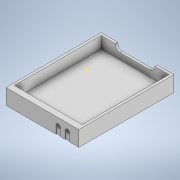
# Autodesk Inventor part: battery-holder-v2
Saved by Autodesk Inventor 2021.2 (Build 252289000, 289)
## iProperties
Created: 2021-03-31
Part Number: battery-holder-v2
Material: Generic
Document SubType Name: Modeling
Designer: ruby
Density: 1 g/cm^3
Appearance: Default
Author: ruby
Autodesk Inventor part; units mm, degrees
ref_plane "YZ Plane" through (0, 0, 0) normal (1, 0, 0) x (0, 1, 0)
ref_plane "XZ Plane" through (0, 0, 0) normal (0, 1, 0) x (-1, 0, 0)
ref_plane "XY Plane" through (0, 0, 0) normal (0, 0, 1) x (1, 0, 0)
sketch "Sketch2" plane through (0, 0, 0) normal (0, 1, 0) x (-1, 0, 0)
  line L0 (11.092548, -17.745585) -> (-22.307452, -17.745585)
  line L1 (-22.307452, -17.745585) -> (-22.307452, 24.254415)
  line L2 (-22.307452, 24.254415) -> (11.092548, 24.254415)
  line L3 (11.092548, 24.254415) -> (11.092548, -17.745585)
  point P0 (0, 0)
  dimension "d2" = 42
  dimension "d3" = 33.4
  constraints: 8 end point, 2 parallel, 1 horizontal, 1 perpendicular
  measures "d2" distance of L2.end L0.start
  measures "d3" distance of L0.start L0.end
sketch "Sketch2 outline for Extrusion1" plane through (0, 0, 0) normal (0, 1, 0) x (-1, 0, 0)
  line L0 (11.092548, -17.745585) -> (11.092548, 24.254415)
  line L1 (-22.307452, -17.745585) -> (11.092548, -17.745585)
  line L2 (-22.307452, 24.254415) -> (-22.307452, -17.745585)
  line L3 (11.092548, 24.254415) -> (-22.307452, 24.254415)
extrude "Extrusion1" add sketch "Sketch2 outline for Extrusion1" along normal blind 6
sketch "Sketch3" plane through (0, 6, 0) normal (0, 1, 0) x (1, 0, 0)
  line L0 (-9.992548, 16.645585) -> (21.207452, 16.645585)
  line L1 (21.207452, 16.645585) -> (21.207452, -23.154415)
  line L2 (21.207452, -23.154415) -> (-9.992548, -23.154415)
  line L3 (-9.992548, -23.154415) -> (-9.992548, 16.645585)
  line L4 (22.307452, 17.745585) -> (-11.092548, 17.745585)
  line L5 (-11.092548, 17.745585) -> (-11.092548, -24.254415)
  line L6 (22.307452, -24.254415) -> (22.307452, 17.745585)
  line L7 (-11.092548, -24.254415) -> (22.307452, -24.254415)
  point P0 (0, 0)
  dimension "d6" = 1.1
  dimension "d7" = 1.1
  dimension "d8" = 1.1
  dimension "d9" = 1.1
  dimension "d10" = 39.8
  constraints: 8 end point, 2 parallel, 1 horizontal, 1 perpendicular
  measures "d6" distance between parallel lines of L4 L0
  measures "d7" distance between parallel lines of L5 L3
  measures "d8" distance between parallel lines of L6 L1
  measures "d9" distance between parallel lines of L7 L2
  measures "d10" distance of L0.end L1.end
sketch "Sketch3 outline for Extrusion2" plane through (0, 6, 0) normal (0, 1, 0) x (1, 0, 0)
  line L0 (-9.992548, 16.645585) -> (-9.992548, -23.154415)
  line L1 (21.207452, 16.645585) -> (-9.992548, 16.645585)
  line L2 (21.207452, -23.154415) -> (21.207452, 16.645585)
  line L3 (-9.992548, -23.154415) -> (21.207452, -23.154415)
extrude "Extrusion2" cut sketch "Sketch3 outline for Extrusion2" against normal blind 4.9
sketch "Sketch4" plane through (0, 0, 0) normal (0, -1, 0) x (1, 0, 0)
  line L0 (22.307452, -17.745585) -> (-11.092548, -17.745585)
  line L1 (-11.092548, -17.745585) -> (-11.092548, 24.254415)
  line L2 (22.307452, -17.745585) -> (-11.092548, -17.745585)
  line L3 (-11.092548, -17.745585) -> (-11.092548, 24.254415)
  line L4 (-11.092548, 24.254415) -> (22.307452, 24.254415)
  line L5 (22.307452, 24.254415) -> (22.307452, -17.745585)
  point P0 (0, 0)
  constraints: 8 end point, 2 parallel, 1 horizontal, 1 perpendicular
sketch "Sketch4 outline for Extrusion3" plane through (0, 0, 0) normal (0, -1, 0) x (1, 0, 0)
  line L0 (22.307452, -17.745585) -> (22.307452, 24.254415)
  line L1 (-11.092548, -17.745585) -> (22.307452, -17.745585)
  line L2 (-11.092548, 24.254415) -> (-11.092548, -17.745585)
  line L3 (22.307452, 24.254415) -> (-11.092548, 24.254415)
extrude "Extrusion3" add sketch "Sketch4 outline for Extrusion3" along normal blind 0.6
sketch "Sketch5" plane through (-11.092548, 6, 24.254415) normal (0, 0, 1) x (1, 0, 0)
  line L0 (33.4, -6.6) -> (33.4, 0) projected
  line L1 (33.4, -6.6) -> (0, -6.6)
  line L2 (0, -6.6) -> (0, -2.5)
  line L3 (0, -2.5) -> (33.4, -2.5)
  line L4 (33.4, -2.5) -> (33.4, -6.6)
  point P0 (11.092548, -6)
  point P1 (33.4, -2.5)
  constraints: 8 end point, 2 parallel, 1 horizontal, 1 perpendicular
sketch "Sketch5 outline for Extrusion4" plane through (-11.092548, 6, 24.254415) normal (0, 0, 1) x (1, 0, 0)
  line L0 (33.4, -2.5) -> (0, -2.5)
  line L1 (33.4, -6.6) -> (33.4, -2.5)
  line L2 (0, -6.6) -> (33.4, -6.6)
  line L3 (0, -2.5) -> (0, -6.6)
extrude "Extrusion4" add sketch "Sketch5 outline for Extrusion4" along normal blind 3
sketch "Sketch6" plane through (21.207452, 6, 23.154415) normal (0, 0, -1) x (-1, 0, 0)
  line L0 (3.6, -0.9) -> (4.9, -0.9)
  line L1 (4.9, -0.9) -> (4.9, -3.9)
  line L2 (4.9, -3.9) -> (3.6, -3.9)
  line L3 (3.6, -3.9) -> (3.6, -0.9)
  line L4 (0, -4.9) -> (31.2, -4.9) projected
  line L5 (5.6, -0.9) -> (6.9, -0.9)
  line L6 (6.9, -0.9) -> (6.9, -3.9)
  line L7 (6.9, -3.9) -> (5.6, -3.9)
  line L8 (5.6, -3.9) -> (5.6, -0.9)
  line L9 (7.6, -0.9) -> (8.9, -0.9)
  line L10 (8.9, -0.9) -> (8.9, -3.9)
  line L11 (8.9, -3.9) -> (7.6, -3.9)
  line L12 (7.6, -3.9) -> (7.6, -0.9)
  point P0 (21.207452, -6)
  point P1 (0, 0)
  dimension "d17" = 3
  dimension "d18" = 1.3
  dimension "d19" = 3.6
  dimension "d20" = 1
  dimension "d23" = 3
  dimension "d24" = 1.3
  dimension "d25" = 3
  dimension "d26" = 1.3
  dimension "d27" = 1
  dimension "d28" = 1
  dimension "d29" = 0.7
  dimension "d30" = 0.7
  constraints: 24 end point, 6 parallel, 3 horizontal, 3 perpendicular
  measures "d17" distance of L0.end L1.end
  measures "d18" distance of L1.end L2.end
  measures "d19" distance from line of point (0, 0) L3
  measures "d20" distance between parallel lines of L2 L4
  measures "d23" distance of L5.end L6.end
  measures "d24" distance of L6.end L8.start
  measures "d25" distance of L9.end L10.end
  measures "d26" distance of L10.end L12.start
  measures "d27" distance between parallel lines of L4 L7
  measures "d28" distance between parallel lines of L4 L11
  measures "d29" distance between parallel lines of L1 L8
  measures "d30" distance between parallel lines of L6 L12
sketch "Sketch7" plane through (-11.092548, 3.5, 24.254415) normal (0, 1, 0) x (1, 0, 0)
  line L0 (0, 0) -> (33.4, 0) projected
  line L1 (0, 42) -> (0, -3) projected
  line L2 (33.4, 0) -> (0, 0)
  line L3 (0, 0) -> (0, -3)
  line L4 (0, -3) -> (33.4, -3)
  line L5 (33.4, -3) -> (33.4, 0)
  point P0 (11.092548, 24.254415)
  constraints: 8 end point, 2 parallel, 1 horizontal, 1 perpendicular
sketch "Sketch7 outline for Extrusion5" plane through (-11.092548, 3.5, 24.254415) normal (0, 1, 0) x (1, 0, 0)
  line L0 (33.4, -3) -> (33.4, 0)
  line L1 (0, -3) -> (33.4, -3)
  line L2 (0, 0) -> (0, -3)
  line L3 (33.4, 0) -> (0, 0)
extrude "Extrusion5" add sketch "Sketch7 outline for Extrusion5" along normal blind 2.5
sketch "Sketch6 outline for Extrusion6" plane through (21.207452, 6, 23.154415) normal (0, 0, -1) x (-1, 0, 0)
  line L0 (7.6, -0.9) -> (7.6, -3.9)
  line L1 (8.9, -0.9) -> (7.6, -0.9)
  line L2 (8.9, -3.9) -> (8.9, -0.9)
  line L3 (7.6, -3.9) -> (8.9, -3.9)
  line L4 (5.6, -0.9) -> (5.6, -3.9)
  line L5 (6.9, -0.9) -> (5.6, -0.9)
  line L6 (6.9, -3.9) -> (6.9, -0.9)
  line L7 (5.6, -3.9) -> (6.9, -3.9)
  line L8 (3.6, -0.9) -> (3.6, -3.9)
  line L9 (4.9, -0.9) -> (3.6, -0.9)
  line L10 (4.9, -3.9) -> (4.9, -0.9)
  line L11 (3.6, -3.9) -> (4.9, -3.9)
extrude "Extrusion6" cut sketch "Sketch6 outline for Extrusion6" against normal through all
sketch "Sketch8" plane through (0, 6, 0) normal (0, 1, 0) x (1, 0, 0)
  point P0 (0, 0)
sketch "Sketch9" plane through (16.307452, 2.1, 23.154415) normal (0, 1, 0) x (1, 0, 0)
  line L0 (1.3, 0) -> (1.3, -4.1)
  line L1 (0, 0) -> (0, -4.1)
  line L2 (1.3, -2.3) -> (0, -2.3)
  line L3 (0, -2.3) -> (0, -2)
  line L4 (0, -2) -> (1.3, -2)
  line L5 (1.3, -2) -> (1.3, -2.3)
  line L6 (0, 0) -> (1.3, 0)
  line L7 (-0.7, -2.311138) -> (-2, -2.311138)
  line L8 (-2, -2.311138) -> (-2, -2.011138)
  line L9 (-2, -2.011138) -> (-0.7, -2.011138)
  line L10 (-0.7, -2.011138) -> (-0.7, -2.311138)
  line L11 (-0.7, 0) -> (-0.7, -4.1)
  line L12 (-2, 0) -> (-0.7, 0)
  line L13 (-2.7, -2.3) -> (-4, -2.3)
  line L14 (-4, -2) -> (-2.7, -2)
  line L15 (-2.7, -2) -> (-2.7, -2.3)
  line L16 (-4, -2.3) -> (-4, -2)
  line L17 (-4, 0) -> (-2.7, 0)
  point P0 (-16.307452, 23.154415)
  point P1 (1.3, -2)
  point P2 (0, -2.3)
  dimension "d33" = 0.3
  dimension "d34" = 2
  dimension "d35" = 0.3
  dimension "d36" = 1.3
  dimension "d37" = 0
  dimension "d38" = 2.01114
  dimension "d39" = 0.3
  dimension "d40" = 1.3
  dimension "d41" = 0
  dimension "d42" = 2
  constraints: 24 end point, 6 parallel, 3 horizontal, 3 perpendicular, 2 point on line
  measures "d33" distance of L4.end L2.start
  measures "d34" distance between parallel lines of L6 L4
  measures "d35" distance of L9.end L7.start
  measures "d36" distance of L9.start L9.end
  measures "d37" distance between parallel lines of L11 L10
  measures "d38" distance between parallel lines of L12 L9
  measures "d39" distance of L14.end L13.start
  measures "d40" distance of L14.start L14.end
  measures "d41" distance from line of L17.end L15
  measures "d42" distance between parallel lines of L17 L14
sketch "Sketch9 outline for Extrusion7" plane through (16.307452, 2.1, 23.154415) normal (0, 1, 0) x (1, 0, 0)
  line L0 (-4, -2) -> (-4, -2.3)
  line L1 (-2.7, -2) -> (-4, -2)
  line L2 (-2.7, -2.3) -> (-2.7, -2)
  line L3 (-4, -2.3) -> (-2.7, -2.3)
  line L4 (-2, -2.011138) -> (-2, -2.311138)
  line L5 (-0.7, -2.011138) -> (-2, -2.011138)
  line L6 (-0.7, -2.311138) -> (-0.7, -2.011138)
  line L7 (-2, -2.311138) -> (-0.7, -2.311138)
  line L8 (1.3, -2) -> (0, -2)
  line L9 (1.3, -2.3) -> (1.3, -2)
  line L10 (0, -2.3) -> (1.3, -2.3)
  line L11 (0, -2) -> (0, -2.3)
extrude "Extrusion7" add sketch "Sketch9 outline for Extrusion7" along normal up to surface (3.9 mm away)
sketch "Sketch10" plane through (0, 6, 0) normal (0, 1, 0) x (1, 0, 0)
  line L0 (17.607452, -25.654415) -> (16.307452, -25.654415)
  line L1 (16.307452, -25.654415) -> (16.307452, -24.654415)
  line L2 (16.307452, -24.654415) -> (17.607452, -24.654415)
  line L3 (17.607452, -24.654415) -> (17.607452, -25.654415)
  line L4 (21.207452, -23.154415) -> (-9.992548, -23.154415)
  line L5 (13.607452, -25.654415) -> (12.307452, -25.654415)
  line L6 (12.307452, -25.654415) -> (12.307452, -24.654415)
  line L7 (12.307452, -24.654415) -> (13.607452, -24.654415)
  line L8 (13.607452, -24.654415) -> (13.607452, -25.654415)
  line L9 (15.607452, -25.654415) -> (14.307452, -25.654415)
  line L10 (14.307452, -25.654415) -> (14.307452, -24.654415)
  line L11 (14.307452, -24.654415) -> (15.607452, -24.654415)
  line L12 (15.607452, -24.654415) -> (15.607452, -25.654415)
  line L13 (13.607452, -25.454415) -> (13.607452, -27.254415)
  point P0 (0, 0)
  point P1 (17.607452, -23.154415)
  point P2 (15.607452, -27.254415)
  dimension "d45" = 1.3
  dimension "d46" = 1
  dimension "d47" = 0
  dimension "d48" = 1.5
  dimension "d49" = 1.3
  dimension "d50" = 1
  dimension "d51" = 1.3
  dimension "d52" = 1
  dimension "d53" = 1.5
  dimension "d54" = 1.5
  dimension "d55" = 0
  dimension "d56" = 0
  constraints: 24 end point, 6 parallel, 3 horizontal, 3 perpendicular
  measures "d45" distance of L1.end L2.end
  measures "d46" distance of L2.end L0.start
  measures "d47" distance from line of point (17.607, -23.154) L3
  measures "d48" distance between parallel lines of L4 L2
  measures "d49" distance of L6.end L8.start
  measures "d50" distance of L8.start L5.start
  measures "d51" distance of L10.end L12.start
  measures "d52" distance of L12.start L9.start
  measures "d53" distance between parallel lines of L4 L11
  measures "d54" distance between parallel lines of L4 L7
  measures "d55" distance between parallel lines of L13 L8
  measures "d56" distance from line of point (15.607, -27.254) L12
sketch "Sketch10 outline for Extrusion8" plane through (0, 6, 0) normal (0, 1, 0) x (1, 0, 0)
  line L0 (13.607452, -24.654415) -> (12.307452, -24.654415)
  line L1 (13.607452, -25.654415) -> (13.607452, -24.654415)
  line L2 (12.307452, -25.654415) -> (13.607452, -25.654415)
  line L3 (12.307452, -24.654415) -> (12.307452, -25.654415)
  line L4 (15.607452, -25.654415) -> (15.607452, -24.654415)
  line L5 (14.307452, -25.654415) -> (15.607452, -25.654415)
  line L6 (14.307452, -24.654415) -> (14.307452, -25.654415)
  line L7 (15.607452, -24.654415) -> (14.307452, -24.654415)
  line L8 (17.607452, -25.654415) -> (17.607452, -24.654415)
  line L9 (16.307452, -25.654415) -> (17.607452, -25.654415)
  line L10 (16.307452, -24.654415) -> (16.307452, -25.654415)
  line L11 (17.607452, -24.654415) -> (16.307452, -24.654415)
extrude "Extrusion8" cut sketch "Sketch10 outline for Extrusion8" against normal blind 1.5
sketch "Sketch11" plane through (-11.092548, 6, 27.254415) normal (0, 0, 1) x (1, 0, 0)
  line L0 (28.7, 0) -> (28.7, -0.9) projected
  line L1 (27.4, -3.9) -> (27.4, -0.9) projected
  line L2 (28.7, -0.9) -> (27.4, -0.9)
  line L3 (27.4, -0.9) -> (27.4, -1.7)
  line L4 (27.4, -1.7) -> (28.7, -1.7)
  line L5 (28.7, -1.7) -> (28.7, -0.9)
  line L6 (26.7, 0) -> (26.7, -0.9) projected
  line L7 (25.4, -3.9) -> (25.4, -1.5) projected
  line L8 (26.7, -0.9) -> (25.4, -0.9)
  line L9 (25.4, -0.9) -> (25.4, -1.7)
  line L10 (25.4, -1.7) -> (26.7, -1.7)
  line L11 (26.7, -1.7) -> (26.7, -0.9)
  line L12 (24.7, -0.9) -> (24.7, -3.9) projected
  line L13 (23.4, -3.9) -> (23.4, -0.9) projected
  line L14 (24.7, -0.9) -> (23.4, -0.9)
  line L15 (23.4, -0.9) -> (23.4, -1.7)
  line L16 (23.4, -1.7) -> (24.7, -1.7)
  line L17 (24.7, -1.7) -> (24.7, -0.9)
  point P0 (11.092548, -6)
  point P1 (24.7, -1.7)
  dimension "d59" = 0.8
  constraints: 24 end point, 6 parallel, 5 point on line, 3 horizontal, 3 perpendicular
  measures "d59" distance of L4.end L0.end
sketch "Sketch11 outline for Extrusion9" plane through (-11.092548, 6, 27.254415) normal (0, 0, 1) x (1, 0, 0)
  line L0 (24.7, -0.9) -> (23.4, -0.9)
  line L1 (24.7, -1.7) -> (24.7, -0.9)
  line L2 (23.4, -1.7) -> (24.7, -1.7)
  line L3 (23.4, -0.9) -> (23.4, -1.7)
  line L4 (26.7, -0.9) -> (25.4, -0.9)
  line L5 (25.4, -0.9) -> (25.4, -1.7)
  line L6 (25.4, -1.7) -> (26.7, -1.7)
  line L7 (26.7, -1.7) -> (26.7, -0.9)
  line L8 (28.7, -0.9) -> (27.4, -0.9)
  line L9 (28.7, -1.7) -> (28.7, -0.9)
  line L10 (27.4, -1.7) -> (28.7, -1.7)
  line L11 (27.4, -0.9) -> (27.4, -1.7)
extrude "Extrusion9" add sketch "Sketch11 outline for Extrusion9" against normal up to surface (1.6 mm away)
sketch "Sketch12" plane through (0, 6, 0) normal (0, 1, 0) x (1, 0, 0)
  line L0 (-11.092548, -27.254415) -> (22.307452, -27.254415)
  line L1 (-11.092548, 17.745585) -> (-11.092548, -27.254415)
  line L2 (22.307452, -27.254415) -> (-11.092548, -27.254415)
  line L3 (-11.092548, -27.254415) -> (-11.092548, -26.754415)
  line L4 (-11.092548, -26.754415) -> (22.307452, -26.754415)
  line L5 (22.307452, -26.754415) -> (22.307452, -27.254415)
  line L6 (17.607452, -25.654415) -> (16.307452, -25.654415)
  point P0 (0, 0)
  dimension "d62" = 1.1
  constraints: 8 end point, 2 parallel, 1 horizontal, 1 perpendicular, 1 point on line
  measures "d62" distance between parallel lines of L6 L4
sketch "Sketch12 outline for Extrusion10" plane through (0, 6, 0) normal (0, 1, 0) x (1, 0, 0)
  line L0 (22.307452, -27.254415) -> (22.307452, -26.754415)
  line L1 (-11.092548, -27.254415) -> (22.307452, -27.254415)
  line L2 (-11.092548, -26.754415) -> (-11.092548, -27.254415)
  line L3 (22.307452, -26.754415) -> (-11.092548, -26.754415)
extrude "Extrusion10" cut sketch "Sketch12 outline for Extrusion10" against normal through all
sketch "Sketch13" plane through (-11.092548, 6, 26.754415) normal (0, 0, 1) x (1, 0, 0)
  line L0 (23.4, -1.7) -> (23.4, -3.9) projected
  line L1 (24.7, -3.9) -> (24.7, -1.7) projected
  line L2 (23.4, -1.7) -> (24.7, -1.7)
  line L3 (24.7, -1.7) -> (24.7, -3.9)
  line L4 (24.7, -3.9) -> (23.4, -3.9)
  line L5 (23.4, -3.9) -> (23.4, -1.7)
  line L6 (26.7, -1.7) -> (25.4, -1.7) projected
  line L7 (25.4, -3.9) -> (26.7, -3.9) projected
  line L8 (25.4, -1.7) -> (26.7, -1.7)
  line L9 (26.7, -1.7) -> (26.7, -3.9)
  line L10 (26.7, -3.9) -> (25.4, -3.9)
  line L11 (25.4, -3.9) -> (25.4, -1.7)
  line L12 (27.4, -3.9) -> (27.4, -1.5) projected
  line L13 (28.7, -3.9) -> (28.7, -0.9) projected
  line L14 (27.4, -1.7) -> (28.7, -1.7)
  line L15 (28.7, -1.7) -> (28.7, -3.9)
  line L16 (28.7, -3.9) -> (27.4, -3.9)
  line L17 (27.4, -3.9) -> (27.4, -1.7)
  point P0 (11.092548, -6)
  point P1 (28.7, -1.7)
  constraints: 24 end point, 6 parallel, 3 horizontal, 3 perpendicular, 2 point on line
sketch "Sketch13 outline for Extrusion11" plane through (-11.092548, 6, 26.754415) normal (0, 0, 1) x (1, 0, 0)
  line L0 (27.4, -3.9) -> (28.7, -3.9)
  line L1 (27.4, -1.7) -> (27.4, -3.9)
  line L2 (28.7, -1.7) -> (27.4, -1.7)
  line L3 (28.7, -3.9) -> (28.7, -1.7)
  line L4 (26.7, -3.9) -> (26.7, -1.7)
  line L5 (25.4, -3.9) -> (26.7, -3.9)
  line L6 (25.4, -1.7) -> (25.4, -3.9)
  line L7 (26.7, -1.7) -> (25.4, -1.7)
  line L8 (24.7, -1.7) -> (23.4, -1.7)
  line L9 (24.7, -3.9) -> (24.7, -1.7)
  line L10 (23.4, -3.9) -> (24.7, -3.9)
  line L11 (23.4, -1.7) -> (23.4, -3.9)
extrude "Extrusion11" cut sketch "Sketch13 outline for Extrusion11" against normal through all
sketch "Sketch14" plane through (0, -0.6, 0) normal (0, -1, 0) x (1, 0, 0)
  point P0 (0, 0)
sketch "Sketch15" plane through (22.307452, 6, -17.745585) normal (0, 0, -1) x (-1, 0, 0)
  line L0 (6, -3.9) -> (6, -1.7) projected
  line L1 (4.7, -3.9) -> (6, -3.9) projected
  line L2 (6, -1.7) -> (4.7, -1.7)
  line L3 (4.7, -1.7) -> (4.7, -3.9)
  line L4 (4.7, -3.9) -> (6, -3.9)
  line L5 (6, -3.9) -> (6, -1.7)
  line L6 (6.7, -1.7) -> (8, -1.7) projected
  line L7 (6.7, -1.7) -> (6.7, -3.9) projected
  line L8 (8, -1.7) -> (6.7, -1.7)
  line L9 (6.7, -1.7) -> (6.7, -3.9)
  line L10 (6.7, -3.9) -> (8, -3.9)
  line L11 (8, -3.9) -> (8, -1.7)
  line L12 (10, -1.7) -> (10, -3.9) projected
  line L13 (8.7, -3.9) -> (10, -3.9) projected
  line L14 (10, -1.7) -> (8.7, -1.7)
  line L15 (8.7, -1.7) -> (8.7, -3.9)
  line L16 (8.7, -3.9) -> (10, -3.9)
  line L17 (10, -3.9) -> (10, -1.7)
  point P0 (22.307452, -6)
  constraints: 24 end point, 6 parallel, 3 horizontal, 3 perpendicular
sketch "Sketch15 outline for Extrusion12" plane through (22.307452, 6, -17.745585) normal (0, 0, -1) x (-1, 0, 0)
  line L0 (8.7, -1.7) -> (8.7, -3.9)
  line L1 (10, -1.7) -> (8.7, -1.7)
  line L2 (10, -3.9) -> (10, -1.7)
  line L3 (8.7, -3.9) -> (10, -3.9)
  line L4 (8, -3.9) -> (8, -1.7)
  line L5 (6.7, -3.9) -> (8, -3.9)
  line L6 (6.7, -1.7) -> (6.7, -3.9)
  line L7 (8, -1.7) -> (6.7, -1.7)
  line L8 (4.7, -1.7) -> (4.7, -3.9)
  line L9 (6, -1.7) -> (4.7, -1.7)
  line L10 (6, -3.9) -> (6, -1.7)
  line L11 (4.7, -3.9) -> (6, -3.9)
extrude "Extrusion12" add sketch "Sketch15 outline for Extrusion12" against normal blind 1.1
sketch "Sketch16" plane through (0, 6, 0) normal (0, 1, 0) x (1, 0, 0)
  line L0 (17.607452, -25.654415) -> (16.307452, -25.654415)
  line L1 (17.607452, -24.654415) -> (16.307452, -24.654415)
  line L2 (16.307452, -25.654415) -> (17.607452, -25.654415)
  line L3 (17.607452, -25.654415) -> (17.607452, -24.654415)
  line L4 (17.607452, -24.654415) -> (16.307452, -24.654415)
  line L5 (16.307452, -24.654415) -> (16.307452, -25.654415)
  line L6 (15.607452, -24.654415) -> (14.307452, -24.654415)
  line L7 (14.307452, -25.654415) -> (15.607452, -25.654415)
  line L8 (15.607452, -25.654415) -> (15.607452, -24.654415)
  line L9 (15.607452, -24.654415) -> (14.307452, -24.654415)
  line L10 (14.307452, -24.654415) -> (14.307452, -25.654415)
  line L11 (13.607452, -25.654415) -> (12.307452, -25.654415)
  line L12 (13.607452, -24.654415) -> (13.607452, -25.654415)
  line L13 (12.307452, -25.654415) -> (13.607452, -25.654415)
  line L14 (13.607452, -25.654415) -> (13.607452, -24.654415)
  line L15 (13.607452, -24.654415) -> (12.307452, -24.654415)
  line L16 (12.307452, -24.654415) -> (12.307452, -25.654415)
  point P0 (0, 0)
  constraints: 24 end point, 6 parallel, 3 horizontal, 3 perpendicular
sketch "Sketch16 outline for Extrusion13" plane through (0, 6, 0) normal (0, 1, 0) x (1, 0, 0)
  line L0 (12.307452, -24.654415) -> (12.307452, -25.654415)
  line L1 (13.607452, -24.654415) -> (12.307452, -24.654415)
  line L2 (13.607452, -25.654415) -> (13.607452, -24.654415)
  line L3 (12.307452, -25.654415) -> (13.607452, -25.654415)
  line L4 (15.607452, -25.654415) -> (15.607452, -24.654415)
  line L5 (14.307452, -25.654415) -> (15.607452, -25.654415)
  line L6 (14.307452, -24.654415) -> (14.307452, -25.654415)
  line L7 (15.607452, -24.654415) -> (14.307452, -24.654415)
  line L8 (17.607452, -25.654415) -> (17.607452, -24.654415)
  line L9 (16.307452, -25.654415) -> (17.607452, -25.654415)
  line L10 (16.307452, -24.654415) -> (16.307452, -25.654415)
  line L11 (17.607452, -24.654415) -> (16.307452, -24.654415)
extrude "Extrusion13" cut sketch "Sketch16 outline for Extrusion13" against normal up to surface (3.9 mm away)
sketch "Sketch17" plane through (0, 6, 0) normal (0, 1, 0) x (1, 0, 0)
  line L0 (22.307452, -26.754415) -> (22.307452, 17.745585)
  line L1 (-11.092548, 17.745585) -> (-11.092548, -26.754415)
  line L2 (22.307452, -26.754415) -> (-11.092548, -26.754415)
  line L3 (-11.092548, -26.754415) -> (-11.092548, -25.654415)
  line L4 (-11.092548, -25.654415) -> (22.307452, -25.654415)
  line L5 (22.307452, -25.654415) -> (22.307452, -26.754415)
  point P0 (0, 0)
  dimension "d71" = 1.1
  constraints: 8 end point, 2 parallel, 1 horizontal, 1 perpendicular, 1 point on line
  measures "d71" distance between parallel lines of L2 L4
sketch "Sketch17 outline for Extrusion14" plane through (0, 6, 0) normal (0, 1, 0) x (1, 0, 0)
  line L0 (-11.092548, -26.754415) -> (22.307452, -26.754415)
  line L1 (-11.092548, -25.654415) -> (-11.092548, -26.754415)
  line L2 (22.307452, -25.654415) -> (-11.092548, -25.654415)
  line L3 (22.307452, -26.754415) -> (22.307452, -25.654415)
extrude "Extrusion14" cut sketch "Sketch17 outline for Extrusion14" against normal through all
sketch "Sketch18" plane through (-11.092548, 6, 25.654415) normal (0, 0, 1) x (1, 0, 0)
  line L0 (27.4, -3.9) -> (28.7, -3.9) projected
  line L1 (32.3, 0) -> (1.1, 0) projected
  line L2 (28.7, -3.9) -> (28.9, -3.9)
  line L3 (28.9, -3.9) -> (28.9, 0)
  line L4 (28.9, 0) -> (28.7, 0)
  line L5 (28.7, 0) -> (28.7, -3.9)
  line L6 (23.4, -3.9) -> (24.7, -3.9) projected
  line L7 (23.4, -3.9) -> (23.2, -3.9)
  line L8 (23.2, -3.9) -> (23.2, 0)
  line L9 (23.2, 0) -> (23.4, 0)
  line L10 (23.4, 0) -> (23.4, -3.9)
  point P0 (11.092548, -6)
  point P1 (23.2, 0)
  dimension "d74" = 0.2
  dimension "d75" = 0.2
  constraints: 16 end point, 4 parallel, 2 horizontal, 2 perpendicular, 2 point on line
  measures "d74" distance of L0.end L2.end
  measures "d75" distance of L6.start L7.end
sketch "Sketch18 outline for Extrusion15" plane through (-11.092548, 6, 25.654415) normal (0, 0, 1) x (1, 0, 0)
  line L0 (23.2, -3.9) -> (23.4, -3.9)
  line L1 (23.2, 0) -> (23.2, -3.9)
  line L2 (23.4, 0) -> (23.2, 0)
  line L3 (23.4, -3.9) -> (23.4, 0)
  line L4 (28.7, -3.9) -> (28.9, -3.9)
  line L5 (28.7, 0) -> (28.7, -3.9)
  line L6 (28.9, 0) -> (28.7, 0)
  line L7 (28.9, -3.9) -> (28.9, 0)
extrude "Extrusion15" cut sketch "Sketch18 outline for Extrusion15" against normal up to surface (1 mm away)
sketch "Sketch19" plane through (-11.092548, -0.6, 25.654415) normal (0, 0, 1) x (1, 0, 0)
  line L0 (28.7, 5.7) -> (27.4, 5.7)
  line L1 (28.9, 2.7) -> (28.9, 6.6)
  line L2 (28.7, 5.7) -> (28.9, 5.7)
  line L3 (28.9, 5.7) -> (28.9, 2.798247)
  line L4 (28.9, 2.798247) -> (28.7, 2.798247)
  line L5 (28.7, 2.798247) -> (28.7, 5.7)
  line L6 (24.7, 5.7) -> (23.4, 5.7)
  line L7 (23.2, 6.6) -> (23.2, 2.7)
  line L8 (23.4, 5.7) -> (23.2, 5.7)
  line L9 (23.2, 5.7) -> (23.2, 2.7)
  line L10 (23.2, 2.7) -> (23.4, 2.7)
  line L11 (23.4, 2.7) -> (23.4, 5.7)
  point P0 (11.092548, 0.6)
  constraints: 16 end point, 4 parallel, 2 horizontal, 2 perpendicular, 1 point on line
sketch "Sketch19 outline for Extrusion16" plane through (-11.092548, -0.6, 25.654415) normal (0, 0, 1) x (1, 0, 0)
  line L0 (28.7, 5.7) -> (28.7, 2.798247)
  line L1 (28.9, 5.7) -> (28.7, 5.7)
  line L2 (28.9, 2.798247) -> (28.9, 5.7)
  line L3 (28.7, 2.798247) -> (28.9, 2.798247)
  line L4 (23.4, 2.7) -> (23.4, 5.7)
  line L5 (23.2, 2.7) -> (23.4, 2.7)
  line L6 (23.2, 5.7) -> (23.2, 2.7)
  line L7 (23.4, 5.7) -> (23.2, 5.7)
extrude "Extrusion16" cut sketch "Sketch19 outline for Extrusion16" against normal up to surface (42.3 mm away)
sketch "Sketch20" plane through (17.607452, 2.1, 24.654415) normal (0, 0, 1) x (1, 0, 0)
  line L0 (0.2, 0) -> (-1.3, 0) projected
  line L1 (-1.3, 3.9) -> (-1.3, 0) projected
  line L2 (0.2, 0) -> (-1.3, 0)
  line L3 (-1.3, 0) -> (-1.3, 3.9)
  line L4 (-1.3, 3.9) -> (0.2, 3.9)
  line L5 (0.2, 3.9) -> (0.2, 0)
  point P0 (-17.607452, -2.1)
  constraints: 8 end point, 2 parallel, 1 horizontal, 1 perpendicular
sketch "Sketch21" plane through (17.607452, 2.1, 24.654415) normal (0, 0, 1) x (1, 0, 0)
  line L0 (0, 0) -> (0, 0.098247)
  line L1 (0.2, 0) -> (-1.3, 0)
  line L2 (0, 0.098247) -> (0.2, 0.098247)
  line L3 (0.2, 0.098247) -> (0.2, 0)
  line L4 (0.2, 0) -> (0, 0)
  line L5 (0, 0) -> (0, 0.098247)
  point P0 (-17.607452, -2.1)
  constraints: 8 end point, 2 parallel, 1 horizontal, 1 perpendicular
sketch "Sketch21 outline for Extrusion17" plane through (17.607452, 2.1, 24.654415) normal (0, 0, 1) x (1, 0, 0)
  line L0 (0.2, 0) -> (0.2, 0.098247)
  line L1 (0, 0) -> (0.2, 0)
  line L2 (0, 0.098247) -> (0, 0)
  line L3 (0.2, 0.098247) -> (0, 0.098247)
extrude "Extrusion17" cut sketch "Sketch21 outline for Extrusion17" against normal blind 2
sketch "Sketch22" plane through (0, 6, 0) normal (0, 1, 0) x (1, 0, 0)
  point P0 (0, 0)
sketch "Sketch23" plane through (-11.092548, -0.6, 25.654415) normal (0, 0, 1) x (1, 0, 0)
  circle A0 centre (28.15, 3.7) radius 1
  line L0 (28.9, 2.7) -> (27.4, 2.7)
  circle A1 centre (23.95, 3.7) radius 1
  line L1 (24.7, 2.7) -> (23.2, 2.7)
  line L2 (23.2, 2.7) -> (23.2, 6.6)
  line L3 (28.9, 6.6) -> (28.9, 2.7)
  line L4 (27.4, 5.7) -> (27.4, 2.7)
  line L5 (28.9, 2.7) -> (27.4, 2.7)
  line L6 (27.4, 2.7) -> (27.4, 3.157237)
  line L7 (27.4, 3.157237) -> (28.9, 3.157237)
  line L8 (28.9, 3.157237) -> (28.9, 2.7)
  line L9 (24.7, 2.7) -> (24.7, 5.7)
  line L10 (23.2, 5.7) -> (23.2, 2.7)
  line L11 (24.7, 2.7) -> (23.2, 2.7)
  line L12 (23.2, 2.7) -> (23.2, 3.216306)
  line L13 (23.2, 3.216306) -> (24.7, 3.216306)
  line L14 (24.7, 3.216306) -> (24.7, 2.7)
  point P0 (11.092548, 0.6)
  point P1 (24.7, 3.216306)
  point P2 (23.2, 3.216306)
  dimension "d82" = 1
  dimension "d83" = 2
  dimension "d84" = 2
  dimension "d85" = 1
  dimension "d86" = 0.75
  constraints: 16 end point, 4 parallel, 2 centre point, 2 horizontal, 2 perpendicular, 2 point on line
  measures "d82" distance from line of L0 A0.centre
  measures "d83" diameter of A0
  measures "d84" diameter of A1
  measures "d85" distance from line of L1 A1.centre
  measures "d86" distance from line of L2 A1.centre
sketch "Sketch23 outline for Extrusion18" plane through (-11.092548, -0.6, 25.654415) normal (0, 0, 1) x (1, 0, 0)
  line L0 (24.7, 3.216306) -> (23.2, 3.216306)
  line L1 (24.7, 2.7) -> (24.7, 3.216306)
  line L2 (23.2, 2.7) -> (24.7, 2.7)
  line L3 (23.2, 3.216306) -> (23.2, 2.7)
  line L4 (27.4, 3.157237) -> (27.4, 2.7)
  line L5 (28.9, 3.157237) -> (27.4, 3.157237)
  line L6 (28.9, 2.7) -> (28.9, 3.157237)
  line L7 (27.4, 2.7) -> (28.9, 2.7)
extrude "Extrusion18" add sketch "Sketch23 outline for Extrusion18" against normal blind 2.5
sketch "Sketch24" plane through (-11.092548, -0.6, 25.654415) normal (0, 0, 1) x (1, 0, 0)
  circle A0 centre (28.15, 3.7) radius 1
  circle A1 centre (23.95, 3.7) radius 1
  line L0 (27.4, 6.6) -> (27.4, 3.157237)
  line L1 (25.4, 2.7) -> (26.7, 2.7)
  line L2 (23.2, 3.216306) -> (23.2, 6.6)
  point P0 (11.092548, 0.6)
  dimension "d89" = 0.75
  dimension "d90" = 2
  dimension "d91" = 1
  dimension "d92" = 0.75
  dimension "d93" = 1
  dimension "d94" = 2
  constraints: 2 centre point
  measures "d89" distance from line of L0 A0.centre
  measures "d90" diameter of A0
  measures "d91" distance from line of L1 A0.centre
  measures "d92" distance from line of L2 A1.centre
  measures "d93" distance from line of L1 A1.centre
  measures "d94" diameter of A1
sketch "Sketch24 outline for Extrusion19" plane through (-11.092548, -0.6, 25.654415) normal (0, 0, 1) x (1, 0, 0)
  circle A0 centre (23.95, 3.7) radius 1
  circle A1 centre (28.15, 3.7) radius 1
extrude "Extrusion19" cut sketch "Sketch24 outline for Extrusion19" against normal blind 0.1
sketch "Sketch25" plane through (-11.092548, -0.6, 25.654415) normal (0, 0, 1) x (1, 0, 0)
  line L0 (28.9, 3.157237) -> (28.9, 5.7)
  line L1 (26.7, 6.6) -> (27.4, 6.6)
  line L2 (28.9, 3.157237) -> (27.4, 3.157237)
  line L3 (27.4, 3.157237) -> (27.4, 6.6)
  line L4 (27.4, 6.6) -> (28.9, 6.6)
  line L5 (28.9, 6.6) -> (28.9, 3.157237)
  line L6 (24.7, 3.216306) -> (24.7, 5.7)
  line L7 (23.2, 6.6) -> (23.2, 5.7)
  line L8 (24.7, 3.216306) -> (23.2, 3.216306)
  line L9 (23.2, 3.216306) -> (23.2, 6.6)
  line L10 (23.2, 6.6) -> (24.7, 6.6)
  line L11 (24.7, 6.6) -> (24.7, 3.216306)
  line L12 (25.4, 2.7) -> (26.7, 2.7)
  line L13 (25.4, 6.6) -> (25.4, 2.7)
  line L14 (26.7, 2.7) -> (25.4, 2.7)
  line L15 (25.4, 2.7) -> (25.4, 6.6)
  line L16 (25.4, 6.6) -> (26.7, 6.6)
  line L17 (26.7, 6.6) -> (26.7, 2.7)
  point P0 (11.092548, 0.6)
  point P1 (28.9, 5.7)
  constraints: 24 end point, 6 parallel, 3 horizontal, 3 perpendicular
sketch "Sketch25 outline for Extrusion20" plane through (-11.092548, -0.6, 25.654415) normal (0, 0, 1) x (1, 0, 0)
  line L0 (23.2, 3.216306) -> (24.7, 3.216306)
  line L1 (24.7, 3.216306) -> (24.7, 6.6)
  line L2 (24.7, 6.6) -> (23.2, 6.6)
  line L3 (23.2, 6.6) -> (23.2, 3.216306)
  line L4 (26.7, 2.7) -> (26.7, 6.6)
  line L5 (25.4, 2.7) -> (26.7, 2.7)
  line L6 (25.4, 6.6) -> (25.4, 2.7)
  line L7 (26.7, 6.6) -> (25.4, 6.6)
  line L8 (28.9, 6.6) -> (27.4, 6.6)
  line L9 (27.4, 6.6) -> (27.4, 3.157237)
  line L10 (27.4, 3.157237) -> (28.9, 3.157237)
  line L11 (28.9, 3.157237) -> (28.9, 6.6)
extrude "Extrusion20" add sketch "Sketch25 outline for Extrusion20" against normal blind 2.5
sketch "Sketch26" plane through (-11.092548, 6, 25.654415) normal (0, 0, 1) x (1, 0, 0)
  arc A0 (27.4, -2.238562) -> (28.9, -2.238562) centre (28.15, -2.9) ccw
  circle A1 centre (28.15, -2.9) radius 0.75
  arc A2 (23.2, -2.238562) -> (24.7, -2.238562) centre (23.95, -2.9) ccw
  circle A3 centre (23.95, -2.9) radius 0.75
  point P0 (11.092548, -6)
  dimension "d99" = 1.5
  dimension "d100" = 1.5
  constraints: 2 centre point, 2 coincident
  measures "d99" diameter of A1
  measures "d100" diameter of A3
sketch "Sketch26 outline for Extrusion21" plane through (-11.092548, 6, 25.654415) normal (0, 0, 1) x (1, 0, 0)
  circle A0 centre (23.95, -2.9) radius 0.75
  circle A1 centre (28.15, -2.9) radius 0.75
extrude "Extrusion21" cut sketch "Sketch26 outline for Extrusion21" against normal blind 2.5
sketch "Sketch27" plane through (-11.092548, 6, 25.654415) normal (0, 0, 1) x (1, 0, 0)
  circle A0 centre (28.15, -2.9) radius 0.75
  circle A1 centre (28.15, -2.9) radius 1
  arc A2 (23.2, -2.238562) -> (24.7, -2.238562) centre (23.95, -2.9) ccw
  circle A3 centre (23.95, -2.9) radius 1
  point P0 (11.092548, -6)
  constraints: 2 centre point, 2 coincident
sketch "Sketch27 outline for Extrusion22" plane through (-11.092548, 6, 25.654415) normal (0, 0, 1) x (1, 0, 0)
  circle A0 centre (23.95, -2.9) radius 1
  circle A1 centre (28.15, -2.9) radius 1
extrude "Extrusion22" cut sketch "Sketch27 outline for Extrusion22" against normal blind 0.1
sketch "Sketch28" plane through (-11.092548, 6, 25.654415) normal (0, 0, 1) x (1, 0, 0)
  line L0 (33.4, 0) -> (33.4, -6.6) projected
  line L1 (33.4, -6.6) -> (0, -6.6)
  line L2 (0, -6.6) -> (0, 0)
  line L3 (0, 0) -> (33.4, 0)
  line L4 (33.4, 0) -> (33.4, -6.6)
  point P0 (11.092548, -6)
  constraints: 8 end point, 2 parallel, 1 horizontal, 1 perpendicular
sketch "Sketch28 outline for Extrusion23" plane through (-11.092548, 6, 25.654415) normal (0, 0, 1) x (1, 0, 0)
  line L0 (33.4, 0) -> (0, 0)
  line L1 (33.4, -6.6) -> (33.4, 0)
  line L2 (0, -6.6) -> (33.4, -6.6)
  line L3 (0, 0) -> (0, -6.6)
extrude "Extrusion23" add sketch "Sketch28 outline for Extrusion23" along normal blind 0.2
sketch "Sketch29" plane through (21.207452, 6, 23.154415) normal (0, 0, -1) x (-1, 0, 0)
  circle A0 centre (4.15, -2.9) radius 0.75 projected
  circle A1 centre (4.15, -2.9) radius 1
  circle A2 centre (8.35, -2.9) radius 0.75 projected
  circle A3 centre (8.35, -2.9) radius 1
  point P0 (21.207452, -6)
  constraints: 2 centre point, 2 coincident
sketch "Sketch30" plane through (-11.092548, 6, 25.854415) normal (0, 0, 1) x (1, 0, 0)
  circle A0 centre (28.15, -2.9) radius 0.75 projected
  circle A1 centre (28.15, -2.9) radius 1
  circle A2 centre (23.95, -2.9) radius 0.75 projected
  circle A3 centre (23.95, -2.9) radius 1
  point P0 (11.092548, -6)
  constraints: 2 centre point, 2 coincident
sketch "Sketch30 outline for Extrusion24" plane through (-11.092548, 6, 25.854415) normal (0, 0, 1) x (1, 0, 0)
  circle A0 centre (23.95, -2.9) radius 1
  circle A1 centre (23.95, -2.9) radius 0.75
  circle A2 centre (28.15, -2.9) radius 1
  circle A3 centre (28.15, -2.9) radius 0.75
extrude "Extrusion24" cut sketch "Sketch30 outline for Extrusion24" against normal blind 0.2
sketch "Sketch29 outline for Extrusion25" plane through (21.207452, 6, 23.154415) normal (0, 0, -1) x (-1, 0, 0)
  circle A0 centre (4.15, -2.9) radius 0.75
  circle A1 centre (8.35, -2.9) radius 0.75
extrude "Extrusion25" cut sketch "Sketch29 outline for Extrusion25" along normal up to surface (39.8 mm away)
sketch "Sketch31" plane through (-11.092548, 6, 25.854415) normal (0, 0, 1) x (1, 0, 0)
  circle A0 centre (28.15, -2.9) radius 0.75 projected
  circle A1 centre (28.15, -2.9) radius 0.75
  circle A2 centre (23.95, -2.9) radius 0.75 projected
  circle A3 centre (23.95, -2.9) radius 0.75
  point P0 (11.092548, -6)
  constraints: 2 centre point, 2 coincident
sketch "Sketch31 outline for Extrusion26" plane through (-11.092548, 6, 25.854415) normal (0, 0, 1) x (1, 0, 0)
  circle A0 centre (23.95, -2.9) radius 0.75
  circle A1 centre (28.15, -2.9) radius 0.75
extrude "Extrusion26" cut sketch "Sketch31 outline for Extrusion26" against normal blind 3
sketch "Sketch32" plane through (0, 6, 0) normal (0, 1, 0) x (1, 0, 0)
  line L0 (15.96333, -24.407005) -> (18.616219, -24.407005)
  line L1 (18.616219, -24.407005) -> (18.616219, -25.008921)
  line L2 (18.616219, -25.008921) -> (15.96333, -25.008921)
  line L3 (15.96333, -25.008921) -> (15.96333, -24.407005)
  point P0 (0, 0)
  constraints: 8 end point, 2 parallel, 1 horizontal, 1 perpendicular
sketch "Sketch32 outline for Extrusion27" plane through (0, 6, 0) normal (0, 1, 0) x (1, 0, 0)
  line L0 (15.96333, -24.407005) -> (15.96333, -25.008921)
  line L1 (18.616219, -24.407005) -> (15.96333, -24.407005)
  line L2 (18.616219, -25.008921) -> (18.616219, -24.407005)
  line L3 (15.96333, -25.008921) -> (18.616219, -25.008921)
extrude "Extrusion27" add sketch "Sketch32 outline for Extrusion27" against normal blind 1
sketch "Sketch33" plane through (0, 6, 0) normal (0, 1, 0) x (1, 0, 0)
  line L0 (22.307452, -25.854415) -> (-11.092548, -25.854415)
  line L1 (-11.092548, 17.745585) -> (-11.092548, -25.854415)
  line L2 (22.307452, -25.854415) -> (-11.092548, -25.854415)
  line L3 (-11.092548, -25.854415) -> (-11.092548, 17.745585)
  line L4 (-11.092548, 17.745585) -> (22.307452, 17.745585)
  line L5 (22.307452, 17.745585) -> (22.307452, -25.854415)
  line L6 (21.207452, 16.645585) -> (21.207452, -23.154415)
  line L7 (-9.992548, -23.154415) -> (-9.992548, 16.645585)
  line L8 (21.207452, -23.154415) -> (-9.992548, -23.154415)
  line L9 (-9.992548, -23.154415) -> (-9.992548, 16.645585)
  line L10 (-9.992548, 16.645585) -> (21.207452, 16.645585)
  line L11 (21.207452, 16.645585) -> (21.207452, -23.154415)
  point P0 (0, 0)
  constraints: 16 end point, 4 parallel, 2 horizontal, 2 perpendicular
sketch "Sketch33 outline for Extrusion28" plane through (0, 6, 0) normal (0, 1, 0) x (1, 0, 0)
  line L0 (22.307452, -25.854415) -> (22.307452, 17.745585)
  line L1 (-11.092548, -25.854415) -> (22.307452, -25.854415)
  line L2 (22.307452, 17.745585) -> (-11.092548, 17.745585)
  line L3 (-11.092548, 17.745585) -> (-11.092548, -25.854415)
  line L4 (21.207452, -23.154415) -> (-9.992548, -23.154415)
  line L5 (21.207452, 16.645585) -> (21.207452, -23.154415)
  line L6 (-9.992548, 16.645585) -> (21.207452, 16.645585)
  line L7 (-9.992548, -23.154415) -> (-9.992548, 16.645585)
extrude "Extrusion28" add sketch "Sketch33 outline for Extrusion28" along normal blind 0.5
sketch "Sketch34" plane through (22.307452, -0.6, -17.745585) normal (0, 0, -1) x (-1, 0, 0)
  line L0 (1.1, 7.1) -> (32.3, 7.1) projected
  line L1 (7.7, 7.1) -> (25.7, 7.1)
  line L2 (25.7, 7.1) -> (25.7, 4.6)
  line L3 (25.7, 4.6) -> (7.7, 4.6)
  line L4 (7.7, 4.6) -> (7.7, 7.1)
  line L5 (0, 0) -> (0, 7.1) projected
  point P0 (22.307452, 0.6)
  point P1 (25.7, 7.1)
  dimension "d117" = 18
  dimension "d118" = 7.7
  dimension "d119" = 2.5
  constraints: 8 end point, 2 parallel, 1 horizontal, 1 perpendicular, 1 point on line
  measures "d117" distance of L2.end L3.end
  measures "d118" distance between parallel lines of L5 L4
  measures "d119" distance of L1.end L2.end
sketch "Sketch34 outline for Extrusion29" plane through (22.307452, -0.6, -17.745585) normal (0, 0, -1) x (-1, 0, 0)
  line L0 (7.7, 4.6) -> (25.7, 4.6)
  line L1 (7.7, 7.1) -> (7.7, 4.6)
  line L2 (25.7, 7.1) -> (7.7, 7.1)
  line L3 (25.7, 4.6) -> (25.7, 7.1)
extrude "Extrusion29" cut sketch "Sketch34 outline for Extrusion29" against normal blind 1.2
fillet "Fillet1" radius 2 2 edges at (-3.3925, 4, -17.1956) (14.6075, 4, -17.1956)
sketch "Sketch35" plane through (-11.092548, 6, 25.854415) normal (0, 0, 1) x (1, 0, 0)
  line L0 (0, -6.6) -> (33.4, -6.6)
  circle A0 centre (28.15, -2.9) radius 1
  line L1 (27.154579, -6.6) -> (29.15, -6.6)
  line L2 (29.15, -6.6) -> (29.15, -2.9)
  line L3 (29.15, -2.9) -> (27.154579, -2.9)
  line L4 (27.154579, -2.9) -> (27.154579, -6.6)
  circle A1 centre (23.95, -2.9) radius 1
  line L5 (22.95, -2.9) -> (24.95, -2.9)
  line L6 (24.95, -2.9) -> (24.95, -6.6)
  line L7 (24.95, -6.6) -> (22.95, -6.6)
  line L8 (22.95, -6.6) -> (22.95, -2.9)
  point P0 (11.092548, -6)
  point P1 (27.154579, -2.995585)
  constraints: 16 end point, 4 parallel, 2 horizontal, 2 perpendicular, 2 point on line, 4 other
sketch "Sketch35 outline for Extrusion30" plane through (-11.092548, 6, 25.854415) normal (0, 0, 1) x (1, 0, 0)
  line L0 (27.154579, -2.995585) -> (27.154579, -6.6)
  arc A0 (29.15, -2.9) -> (27.154579, -2.995585) centre (28.15, -2.9) cw
  line L1 (29.15, -6.6) -> (29.15, -2.9)
  line L2 (27.154579, -6.6) -> (29.15, -6.6)
  line L3 (22.95, -2.9) -> (22.95, -6.6)
  arc A1 (24.95, -2.9) -> (22.95, -2.9) centre (23.95, -2.9) cw
  line L4 (24.95, -6.6) -> (24.95, -2.9)
  line L5 (22.95, -6.6) -> (24.95, -6.6)
extrude "Extrusion30" cut sketch "Sketch35 outline for Extrusion30" against normal blind 0.3
sketch "Sketch36" plane through (0, 6.5, 0) normal (0, 1, 0) x (1, 0, 0)
  point P0 (0, 0)
sketch "Sketch37" plane through (0, 6.5, 0) normal (0, 1, 0) x (1, 0, 0)
  point P0 (0, 0)
sketch "Sketch38" plane through (-11.092548, 6, 25.854415) normal (0, 0, 1) x (1, 0, 0)
  circle A0 centre (28.15, -2.9) radius 0.75 projected
  circle A1 centre (28.15, -2.9) radius 1
  circle A2 centre (23.95, -2.9) radius 0.75 projected
  circle A3 centre (23.95, -2.9) radius 1
  point P0 (11.092548, -6)
  dimension "d125" = 2
  constraints: 2 centre point, 2 coincident
  measures "d125" diameter of A1
sketch "Sketch38 outline for Extrusion31" plane through (-11.092548, 6, 25.854415) normal (0, 0, 1) x (1, 0, 0)
  circle A0 centre (23.95, -2.9) radius 1
  circle A1 centre (23.95, -2.9) radius 0.75
  circle A2 centre (28.15, -2.9) radius 1
  circle A3 centre (28.15, -2.9) radius 0.75
extrude "Extrusion31" cut sketch "Sketch38 outline for Extrusion31" against normal blind 0.6
body "Solid1"
